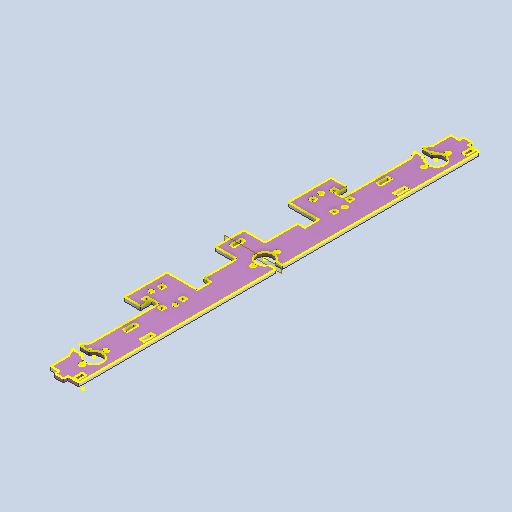
# Autodesk Inventor part: chassis_1_1-03
Saved by Autodesk Inventor 2022 (Build 260153000, 153)
## iProperties
Created: 2023-03-24
Part Number: chassis_1_1-03
Material: 一般
Document SubType Name: Modeling
Designer: Johnny Jou
Density: 79.16 g/cm^3
Appearance: 預設
Mass: 1181.55 g
Surface Area: 130.252 cm^2
Volume: 14.9262 cm^3
Author: Johnny Jou
Autodesk Inventor part; units mm, degrees
ref_plane "YZ Plane" through (0, 0, 0) normal (1, 0, 0) x (0, 1, 0)
ref_plane "XZ Plane" through (0, 0, 0) normal (0, 1, 0) x (-1, 0, 0)
ref_plane "XY Plane" through (0, 0, 0) normal (0, 0, 1) x (1, 0, 0)
sketch "草圖1" plane through (0, 0, 0) normal (0, 1, 0) x (-1, 0, 0)
  line L0 (0, 0) -> (0, -290)
  arc A0 (15, -157.4599) -> (15, -132.5401) centre (16, -145) ccw
  circle A1 centre (16, -145) radius 26 construction
  line L1 (15, -280) -> (15, -157.4599)
  line L2 (15, -132.5401) -> (15, -10)
  circle A2 centre (16, -136.5) radius 1.5
  circle A3 centre (16, -153.5) radius 1.5
  line L3 (20, 0) -> (20, -10)
  line L4 (20, -10) -> (15, -10)
  line L5 (0, -10) -> (0, 0)
  line L6 (6, 0) -> (6, -3)
  line L7 (6, -3) -> (14, -3)
  line L8 (14, -3) -> (14, 0)
  line L9 (0, 0) -> (6, 0)
  line L10 (14, 0) -> (20, 0)
  line L11 (15, 0) -> (14, 0)
  line L12 (6, 0) -> (0, 0)
  line L13 (20, -290) -> (20, -280)
  line L14 (20, -280) -> (15, -280)
  line L15 (0, -290) -> (0, -290)
  line L16 (6, -290) -> (6, -287)
  line L17 (6, -287) -> (14, -287)
  line L18 (14, -287) -> (14, -290)
  line L19 (0, -290) -> (6, -290)
  line L20 (14, -290) -> (20, -290)
  dimension "d1" = 15
  dimension "d2" = 25
  dimension "d3" = 52
  dimension "d4" = 16
  dimension "d6" = 3
  dimension "d7" = 17
  dimension "d8" = 8.5
  dimension "d9" = 10
  dimension "d10" = 20
  dimension "d11" = 8
  dimension "d12" = 3
  dimension "d13" = 6
  dimension "d15" = 3
  dimension "d16" = 8
  dimension "d17" = 6
  dimension "d34" = 290
  dimension "d35" = 145
  dimension "d36" = 10
  dimension "d55" = 8.5
  dimension "d56" = 15
  dimension "d57" = 15
  constraints: 42 end point, 10 parallel, 6 horizontal, 6 perpendicular, 4 centre point, 2 coincident, 2 collinear, 2 point on circle, 1 equal radius, 1 vertical alignment
  measures "d1" distance of L11.start L0.start
  measures "d2" diameter of A0
  measures "d3" diameter of A1
  measures "d4" distance from line of L0 A0.centre
  measures "d6" diameter of A2
  measures "d7" distance of A3.centre A2.centre
  measures "d8" distance of A0.centre A3.centre
  measures "d9" distance of L3.start L3.end
  measures "d10" distance between parallel lines of L0 L3
  measures "d11" distance of L6.end L7.end
  measures "d12" distance of L7.end L8.end
  measures "d13" distance between parallel lines of L5 L6
  measures "d15" distance of L17.end L18.end
  measures "d16" distance of L16.end L17.end
  measures "d17" distance between parallel lines of L0 L16
  measures "d34" distance of L0.start L0.end
  measures "d35" distance from line of L19 A0.centre
  measures "d36" distance of L13.start L13.end
  measures "d55" distance of A0.centre A2.centre
  measures "d56" distance between parallel lines of L0 L1
  measures "d57" distance between parallel lines of L0 L2
extrude "擠出1" add sketch "草圖1" along normal blind 3
sketch "草圖2" plane through (0, 3, 0) normal (0, 1, 0) x (1, 0, 0)
  line L0 (-5, 197) -> (-2, 197)
  line L1 (-2, 197) -> (-2, 205)
  line L2 (-2, 205) -> (-5, 205)
  line L3 (-5, 205) -> (-5, 197)
  arc A0 (-15, 157.4599) -> (-15, 132.5401) centre (-16, 145) ccw projected
  line L4 (-15, 132.5401) -> (-15, 10) projected
  circle A1 centre (-16, 145) radius 12.5 construction
  line L5 (0, 0) -> (0, 290) projected
  line L6 (-11, 4) -> (-8, 4)
  line L7 (-8, 4) -> (-8, 10)
  line L8 (-8, 10) -> (-11, 10)
  line L9 (-11, 10) -> (-11, 4)
  line L10 (-14, 3) -> (-6, 3) projected
  line L11 (-11, 280) -> (-8, 280)
  line L12 (-8, 280) -> (-8, 286)
  line L13 (-8, 286) -> (-11, 286)
  line L14 (-11, 286) -> (-11, 280)
  line L15 (-6, 287) -> (-14, 287) projected
  line L16 (-5, 85) -> (-2, 85)
  line L17 (-2, 85) -> (-2, 93)
  line L18 (-2, 93) -> (-5, 93)
  line L19 (-5, 93) -> (-5, 85)
  line L20 (-15, 280) -> (-15, 157.4599) projected
  line L21 (-13, 129) -> (-5, 129)
  line L22 (-5, 129) -> (-5, 132)
  line L23 (-5, 132) -> (-13, 132)
  line L24 (-13, 132) -> (-13, 129)
  line L25 (-13, 158) -> (-5, 158)
  line L26 (-5, 158) -> (-5, 161)
  line L27 (-5, 161) -> (-13, 161)
  line L28 (-13, 161) -> (-13, 158)
  line L29 (-11, 51) -> (-8, 51)
  line L30 (-8, 51) -> (-8, 59)
  line L31 (-8, 59) -> (-11, 59)
  line L32 (-11, 59) -> (-11, 51)
  line L33 (-11, 55) -> (-8, 55) construction
  line L34 (-11, 231) -> (-8, 231)
  line L35 (-8, 231) -> (-8, 239)
  line L36 (-8, 239) -> (-11, 239)
  line L37 (-11, 239) -> (-11, 231)
  line L38 (-11, 235) -> (-8, 235) construction
  dimension "d20" = 8
  dimension "d21" = 3
  dimension "d22" = 60
  dimension "d23" = 2
  dimension "d24" = 6
  dimension "d25" = 3
  dimension "d27" = 1
  dimension "d28" = 6
  dimension "d29" = 3
  dimension "d31" = 1
  dimension "d58" = 3
  dimension "d59" = 8
  dimension "d60" = 60
  dimension "d69" = 4
  dimension "d70" = 4
  dimension "d104" = 13
  dimension "d106" = 13
  dimension "d108" = 90
  dimension "d109" = 90
  constraints: 68 end point, 16 parallel, 8 equal length, 8 horizontal, 8 perpendicular, 5 collinear, 4 midpoint, 1 coincident, 3 other
  measures "d20" distance of L2.end L0.start
  measures "d21" distance of L1.end L2.end
  measures "d22" distance from line of A0.centre L2
  measures "d23" distance between parallel lines of L5 L1
  measures "d24" distance of L8.end L6.start
  measures "d25" distance of L7.end L8.end
  measures "d27" distance between parallel lines of L10 L6
  measures "d28" distance of L13.end L11.start
  measures "d29" distance of L11.start L11.end
  measures "d31" distance between parallel lines of L15 L13
  measures "d58" distance of L17.end L18.end
  measures "d59" distance of L16.end L17.end
  measures "d60" distance from line of A0.centre L16
  measures "d69" distance between parallel lines of L20 L14
  measures "d70" distance between parallel lines of L4 L9
  measures "d104" distance from line of A0.centre L23
  measures "d106" distance from line of L25 A0.centre
  measures "d108" distance from line of A0.centre L33
  measures "d109" distance from line of A0.centre L38
extrude "擠出2" cut sketch "草圖2" against normal up to surface (3 mm away) contours L9 L8 L7 L6 | L14 L13 L12 L11 | L32 L31 L30 L29 | L37 L36 L35 L34
sketch "草圖3" plane through (0, 3, 0) normal (0, 1, 0) x (1, 0, 0)
  arc A0 (-15, 157.4599) -> (-15, 132.5401) centre (-16, 145) ccw projected
  circle A1 centre (-16, 145) radius 6
  point P0 (0, 0)
  dimension "d37" = 12
  constraints: 1 centre point, 1 coincident
  measures "d37" diameter of A1
extrude "擠出3" cut sketch "草圖3" against normal up to surface (3 mm away)
sketch "草圖4" plane through (0, 3, 0) normal (0, 1, 0) x (1, 0, 0)
  circle A0 centre (-16, 145) radius 6 projected
  arc A1 (-15, 157.4599) -> (-15, 132.5401) centre (-16, 145) ccw projected
  circle A2 centre (-16, 136.5) radius 1.5 projected
  circle A3 centre (-16, 153.5) radius 1.5 projected
  circle A4 centre (-16, 23.5) radius 12.5
  circle A5 centre (-16, 23.5) radius 6
  circle A6 centre (-16, 32) radius 1.5
  circle A7 centre (-16, 15) radius 1.5
  line L0 (-15, 132.5401) -> (-15, 10) projected
  circle A8 centre (-16, 266.5) radius 12.5
  circle A9 centre (-16, 266.5) radius 6
  circle A10 centre (-16, 275) radius 1.5
  circle A11 centre (-16, 258) radius 1.5
  point P0 (0, 0)
  point P1 (-15, 11.0401)
  point P2 (-15, 35.9599)
  dimension "d40" = 3
  dimension "d41" = 12
  dimension "d42" = 25
  dimension "d43" = 17
  dimension "d44" = 8.5
  dimension "d45" = 121.5
  dimension "d48" = 243
  constraints: 8 centre point, 3 vertical alignment, 2 coincident, 1 equal radius, 1 vertical, 8 other
  measures "d40" diameter of A6
  measures "d41" diameter of A5
  measures "d42" diameter of A4
  measures "d43" distance of A7.centre A6.centre
  measures "d44" distance of A4.centre A6.centre
  measures "d45" distance of A0.centre A4.centre
  measures "d48" distance of A4.centre A8.centre
extrude "擠出4" add sketch "草圖4" against normal up to surface (3 mm away) contours A4 L0 A7 A5 A6 | L0 A6 A5 A7 A4 | A8
sketch "草圖6" plane through (0, 3, 0) normal (0, 1, 0) x (1, 0, 0)
  arc A0 (-15, 29.4161) -> (-15, 17.5839) centre (-16, 23.5) ccw projected
  arc A1 (-15, 272.4161) -> (-15, 260.5839) centre (-16, 266.5) ccw projected
  line L0 (-15, 272.4161) -> (-15, 260.5839) projected
  circle A2 centre (-16, 266.5) radius 6
  line L1 (-15, 29.4161) -> (-15, 17.5839) projected
  circle A3 centre (-16, 23.5) radius 6
  point P0 (0, 0)
  point P1 (-15, 260.5839)
  point P2 (-15, 29.4161)
  constraints: 2 coincident, 6 other
extrude "擠出" cut sketch "草圖6" against normal up to surface (3 mm away) contours A3 L1 | L0 A1 | A2 L0
sketch "草圖8" plane through (0, 3, 0) normal (0, 1, 0) x (1, 0, 0)
  circle A0 centre (-16, 266.5) radius 6 projected
  circle A1 centre (-16, 23.5) radius 6 projected
  line L0 (-15, 259.118) -> (-15, 256.882) projected
  arc A2 (-15, 259.118) -> (-15, 256.882) centre (-16, 258) ccw projected
  line L1 (0, 0) -> (0, 290) projected
  line L2 (-6, 290) -> (-6, 287) projected
  line L3 (-6, 287) -> (-14, 287) projected
  line L4 (-14, 287) -> (-14, 290) projected
  line L5 (-14, 290) -> (-20, 290) projected
  line L6 (-20, 290) -> (-20, 280) projected
  line L7 (-20, 280) -> (-15, 280) projected
  line L8 (-15, 280) -> (-15, 278.9599) projected
  arc A3 (-15, 278.9599) -> (-15, 254.0401) centre (-16, 266.5) ccw projected
  line L9 (-15, 254.0401) -> (-15, 157.4599) projected
  arc A4 (-15, 157.4599) -> (-15, 132.5401) centre (-16, 145) ccw projected
  line L10 (-15, 132.5401) -> (-15, 35.9599) projected
  arc A5 (-15, 35.9599) -> (-15, 11.0401) centre (-16, 23.5) ccw projected
  line L11 (-20, 10) -> (-20, 0) projected
  line L12 (-20, 0) -> (-14, 0) projected
  line L13 (-14, 0) -> (-14, 3) projected
  line L14 (-14, 3) -> (-6, 3) projected
  line L15 (-6, 3) -> (-6, 0) projected
  arc A6 (-15, 33.118) -> (-15, 30.882) centre (-16, 32) ccw projected
  line L16 (-15, 33.118) -> (-15, 30.882) projected
  circle A7 centre (-16, 145) radius 6 projected
  line L17 (-8, 286) -> (-8, 280) projected
  line L18 (-8, 280) -> (-11, 280) projected
  line L19 (-11, 280) -> (-11, 286) projected
  line L20 (-11, 286) -> (-8, 286) projected
  line L21 (-8, 4) -> (-11, 4) projected
  line L22 (-11, 4) -> (-11, 10) projected
  line L23 (-8, 10) -> (-8, 4) projected
  circle A8 centre (-16, 136.5) radius 1.5 projected
  circle A9 centre (-16, 153.5) radius 1.5 projected
  arc A10 (-15, 276.118) -> (-15, 273.882) centre (-16, 275) ccw projected
  line L24 (-15, 276.118) -> (-15, 273.882) projected
  circle A11 centre (-20, 40.5367) radius 5
  line L25 (-15, 132.5401) -> (-15, 35.9599) projected
  circle A12 centre (-22.4706, 10) radius 2.4706
  circle A13 centre (-20, 127.9633) radius 5
  circle A14 centre (-20, 162.0367) radius 5
  circle A15 centre (-20, 249.4633) radius 5
  arc A16 (-15, 35.9599) -> (-15, 11.0401) centre (-16, 23.5) ccw projected
  line L26 (-20, 10) -> (-20, 0) projected
  arc A17 (-15, 157.4599) -> (-15, 132.5401) centre (-16, 145) ccw projected
  line L27 (-15, 254.0401) -> (-15, 157.4599) projected
  circle A18 centre (-22.4706, 280) radius 2.4706
  line L28 (-20, 290) -> (-20, 280) projected
  line L29 (-11, 10) -> (-8, 10) projected
  line L30 (-15, 11.0401) -> (-15, 10) projected
  line L31 (-15, 10) -> (-20, 10) projected
  line L32 (0, 290) -> (-6, 290) projected
  line L33 (-6, 0) -> (0, 0) projected
  point P0 (-21.4028, 277.7721)
  point P1 (-18.8571, 254.3309)
  point P2 (-15, 249.4633)
  point P3 (-15, 162.0367)
  point P4 (-18.8571, 157.1691)
  point P5 (-18.8571, 132.8309)
  point P6 (-15, 127.9633)
  point P7 (-15, 40.5367)
  point P8 (-18.8571, 35.6691)
  point P9 (-21.4028, 12.2279)
  point P10 (-20, 9.6573)
  point P11 (-20, 4.6573)
  point P12 (-27.9283, 17.763)
  dimension "d71" = 10
  constraints: 8 tangent, 4 centre point, 3 equal radius, 2 vertical, 8 other
  measures "d71" diameter of A11
extrude "擠出6" add sketch "草圖8" against normal up to surface (3 mm away) contours A12 A5 L30 L31 | L7 L8 A3 A18 | A11 L10 A5 | A3 L9 A15 | A13 A4 L10 | L9 A4 A14
sketch "草圖9" plane through (0, 3, 0) normal (0, 1, 0) x (1, 0, 0)
  circle A0 centre (-16, 266.5) radius 6 projected
  circle A1 centre (-16, 23.5) radius 6 projected
  line L0 (-15, 259.118) -> (-15, 256.882) projected
  arc A2 (-15, 259.118) -> (-15, 256.882) centre (-16, 258) ccw projected
  line L1 (0, 0) -> (0, 290) projected
  line L2 (-6, 290) -> (-6, 287) projected
  line L3 (-6, 287) -> (-14, 287) projected
  line L4 (-14, 287) -> (-14, 290) projected
  line L5 (-14, 290) -> (-20, 290) projected
  line L6 (-20, 290) -> (-20, 280) projected
  arc A3 (-21.4028, 277.7721) -> (-20, 280) centre (-22.4706, 280) ccw projected
  arc A4 (-21.4028, 277.7721) -> (-18.8571, 254.3309) centre (-16, 266.5) ccw projected
  arc A5 (-15, 249.4633) -> (-18.8571, 254.3309) centre (-20, 249.4633) ccw projected
  line L7 (-15, 249.4633) -> (-15, 162.0367) projected
  arc A6 (-18.8571, 157.1691) -> (-15, 162.0367) centre (-20, 162.0367) ccw projected
  arc A7 (-18.8571, 157.1691) -> (-18.8571, 132.8309) centre (-16, 145) ccw projected
  arc A8 (-15, 127.9633) -> (-18.8571, 132.8309) centre (-20, 127.9633) ccw projected
  line L8 (-15, 127.9633) -> (-15, 40.5367) projected
  arc A9 (-18.8571, 35.6691) -> (-15, 40.5367) centre (-20, 40.5367) ccw projected
  arc A10 (-18.8571, 35.6691) -> (-21.4028, 12.2279) centre (-16, 23.5) ccw projected
  arc A11 (-20, 10) -> (-21.4028, 12.2279) centre (-22.4706, 10) ccw projected
  line L9 (-20, 10) -> (-20, 0) projected
  line L10 (-20, 0) -> (-14, 0) projected
  line L11 (-14, 0) -> (-14, 3) projected
  line L12 (-14, 3) -> (-6, 3) projected
  line L13 (-6, 3) -> (-6, 0) projected
  arc A12 (-15, 33.118) -> (-15, 30.882) centre (-16, 32) ccw projected
  line L14 (-15, 33.118) -> (-15, 30.882) projected
  circle A13 centre (-16, 145) radius 6 projected
  line L15 (-8, 286) -> (-8, 280) projected
  line L16 (-8, 280) -> (-11, 280) projected
  line L17 (-11, 280) -> (-11, 286) projected
  line L18 (-11, 286) -> (-8, 286) projected
  line L19 (-8, 4) -> (-11, 4) projected
  line L20 (-11, 4) -> (-11, 10) projected
  line L21 (-8, 10) -> (-8, 4) projected
  circle A14 centre (-16, 136.5) radius 1.5 projected
  circle A15 centre (-16, 153.5) radius 1.5 projected
  arc A16 (-15, 276.118) -> (-15, 273.882) centre (-16, 275) ccw projected
  line L22 (-15, 276.118) -> (-15, 273.882) projected
  arc A17 (-15, 16.118) -> (-15, 13.882) centre (-16, 15) ccw projected
  circle A18 centre (-16, 15) radius 1.5
  line L23 (-15, 33.118) -> (-15, 30.882) projected
  circle A19 centre (-16, 32) radius 1.5
  circle A20 centre (-16, 258) radius 1.5
  circle A21 centre (-16, 275) radius 1.5
  line L24 (-28.5, 264) -> (-21.4544, 264)
  line L25 (-21.4544, 264) -> (-21.4544, 269)
  line L26 (-21.4544, 269) -> (-28.5, 269)
  line L27 (-28.5, 269) -> (-28.5, 264)
  circle A22 centre (-16, 266.5) radius 6 projected
  arc A23 (-21.4028, 277.7721) -> (-18.8571, 254.3309) centre (-16, 266.5) ccw projected
  line L28 (-28.5, 142.5) -> (-21.4544, 142.5)
  line L29 (-21.4544, 142.5) -> (-21.4544, 147.5)
  line L30 (-21.4544, 147.5) -> (-28.5, 147.5)
  line L31 (-28.5, 147.5) -> (-28.5, 142.5)
  circle A24 centre (-16, 145) radius 6 projected
  line L32 (-28.5, 21) -> (-21.4544, 21)
  line L33 (-21.4544, 21) -> (-21.4544, 26)
  line L34 (-21.4544, 26) -> (-28.5, 26)
  line L35 (-28.5, 26) -> (-28.5, 21)
  arc A25 (-18.8571, 35.6691) -> (-21.4028, 12.2279) centre (-16, 23.5) ccw projected
  circle A26 centre (-16, 23.5) radius 6 projected
  line L36 (-11, 10) -> (-8, 10) projected
  line L37 (-15, 16.118) -> (-15, 13.882) projected
  arc A27 (-15, 16.118) -> (-15, 13.882) centre (-16, 15) ccw projected
  line L38 (0, 290) -> (-6, 290) projected
  line L39 (-6, 0) -> (0, 0) projected
  circle A28 centre (-16, 145) radius 6 projected
  line L40 (0, 0) -> (0, 290) projected
  line L41 (-10.5456, 142.5) -> (0, 142.5)
  line L42 (0, 142.5) -> (0, 147.5)
  line L43 (0, 147.5) -> (-10.5456, 147.5)
  line L44 (-10.5456, 147.5) -> (-10.5456, 142.5)
  point P0 (-28.2474, 269)
  point P1 (-28.2474, 264)
  point P2 (-28.2474, 147.5)
  point P3 (-28.2474, 142.5)
  point P4 (-28.2474, 26)
  point P5 (-28.2474, 21)
  point P6 (-15, 30.882)
  point P7 (-21.8029, 14.9747)
  point P8 (-20.38, 12.3993)
  point P9 (-21.4544, 19)
  point P10 (-21.4544, 14.5244)
  point P11 (0, 147.5)
  point P12 (-10.5456, 147.5)
  point P13 (0, 142.5)
  dimension "d74" = 5
  dimension "d75" = 5
  dimension "d76" = 5
  constraints: 32 end point, 8 parallel, 4 coincident, 4 horizontal, 4 perpendicular, 3 point on circle, 3 tangent, 2 collinear, 1 point on line, 20 other
  measures "d74" distance of L26.end L24.start
  measures "d75" distance of L30.end L28.start
  measures "d76" distance of L34.end L32.start
extrude "擠出7" cut sketch "草圖9" against normal up to surface (3 mm away) contours A0 L24 A4 L26 | L43 L1 L41 A13 | L34 A1 L32 A10 | A10 L35 L34 | A10 L32 L35 | A20 L0 | A19 L14 | A21 L22 | L37 A17 | A18 L37
fillet "圓角1" radius 0.5 8 edges at (-21.4544, 1.5, -269) (-28.2474, 1.5, -269) (-21.4544, 1.5, -264) (-28.2474, 1.5, -264) (-21.4544, 1.5, -26) (-28.2474, 1.5, -26) (-28.2474, 1.5, -21) (-21.4544, 1.5, -21)
sketch "草圖11" plane through (0, 3, 0) normal (0, 1, 0) x (1, 0, 0)
  line L0 (-15, 127.9633) -> (-15, 40.5367) projected
  line L1 (-15, 249.4633) -> (-15, 162.0367) projected
  line L2 (-28.5, 242.5) -> (-15, 242.5)
  line L3 (-28.5, 245.5) -> (-28.5, 242.5)
  line L4 (-33.5, 242.5) -> (-28.5, 245.5)
  line L5 (-15, 227.5) -> (-28.5, 227.5)
  line L6 (-28.5, 227.5) -> (-28.5, 224.5)
  line L7 (-33.5, 227.5) -> (-33.5, 242.5)
  line L8 (-28.5, 224.5) -> (-33.5, 227.5)
  arc A0 (-21.3227, 263.7308) -> (-21.3227, 269.2692) centre (-16, 266.5) ccw projected
  arc A1 (-10.5456, 147.5) -> (-10.5456, 142.5) centre (-16, 145) ccw projected
  line L9 (-16, 145) -> (0, 145)
  line L10 (-28.5, 47.5) -> (-15, 47.5)
  line L11 (-28.5, 44.5) -> (-28.5, 47.5)
  line L12 (-33.5, 47.5) -> (-28.5, 44.5)
  line L13 (-15, 62.5) -> (-28.5, 62.5)
  line L14 (-28.5, 62.5) -> (-28.5, 65.5)
  line L15 (-33.5, 62.5) -> (-33.5, 47.5)
  line L16 (-28.5, 65.5) -> (-33.5, 62.5)
  line L17 (-28, 245.5) -> (-15, 245.5)
  line L18 (-15, 245.5) -> (-15, 242.5)
  line L19 (-15, 242.5) -> (-19.5, 242.5)
  line L20 (-28, 243) -> (-28, 245.5)
  line L21 (-15, 227.5) -> (-19.5, 227.5)
  line L22 (-28, 227) -> (-28, 224.5)
  line L23 (-28, 224.5) -> (-15, 224.5)
  line L24 (-15, 224.5) -> (-15, 227.5)
  line L25 (-19.5, 242.5) -> (-27.5, 242.5)
  line L26 (-27.5, 242.5) -> (-27.5, 243)
  line L27 (-27.5, 243) -> (-28, 243)
  line L28 (-19.5, 227.5) -> (-27.5, 227.5)
  line L29 (-27.5, 227.5) -> (-27.5, 227)
  line L30 (-27.5, 227) -> (-28, 227)
  line L31 (-28, 47) -> (-28, 44.5)
  line L32 (-28, 44.5) -> (-15, 44.5)
  line L33 (-27.5, 47.5) -> (-27.5, 47)
  line L34 (-27.5, 47) -> (-28, 47)
  line L35 (-28, 65.5022) -> (-15, 65.5022)
  line L36 (-28, 63.0022) -> (-28, 65.5022)
  line L37 (-27.5, 62.5) -> (-27.5, 63)
  line L38 (-27.5, 63) -> (-28, 63.0022)
  arc A2 (-21.3227, 20.7308) -> (-21.3227, 26.2692) centre (-16, 23.5) ccw projected
  line L39 (-15, 54) -> (-15, 62)
  line L40 (-8, 51) -> (-11, 51) projected
  line L41 (-11, 59) -> (-8, 59) projected
  line L42 (-15, 234) -> (-15, 242)
  line L43 (-8, 231) -> (-11, 231) projected
  line L44 (-11, 239) -> (-8, 239) projected
  line L45 (-22.9, 239) -> (-20, 239)
  line L46 (-20, 239) -> (-20, 231)
  line L47 (-20, 231) -> (-22.9, 231)
  line L48 (-22.9, 231) -> (-22.9, 239)
  line L49 (-8, 239) -> (-11, 239) projected
  line L50 (-11, 231) -> (-8, 231) projected
  line L51 (-11, 239) -> (-11, 231) projected
  line L52 (-22.9, 59) -> (-20, 59)
  line L53 (-20, 59) -> (-20, 51)
  line L54 (-20, 51) -> (-22.9, 51)
  line L55 (-22.9, 51) -> (-22.9, 59)
  line L56 (-8, 59) -> (-11, 59) projected
  line L57 (-11, 51) -> (-8, 51) projected
  line L58 (-11, 59) -> (-11, 51) projected
  point P0 (0, 0)
  point P1 (-22, 148)
  point P2 (-22, 148)
  point P3 (-15, 47.5)
  point P4 (-15, 62.5)
  point P5 (-15, 245.5)
  point P6 (-15, 224.5)
  dimension "d2" = 25
  dimension "d80" = 15
  dimension "d81" = 3
  dimension "d82" = 13.5
  dimension "d83" = 3
  dimension "d84" = 13.5
  dimension "d85" = 24
  dimension "d88" = 5
  dimension "d89" = 0.5
  dimension "d90" = 0.5
  dimension "d91" = 0.5
  dimension "d92" = 0.5
  dimension "d93" = 0.5
  dimension "d94" = 0.5
  dimension "d95" = 0.5
  dimension "d96" = 0.5
  dimension "d97" = 3
  dimension "d98" = 3
  dimension "d99" = 0.5
  dimension "d100" = 0.5
  dimension "d101" = 13
  dimension "d102" = 2.5
  dimension "d103" = 0.5
  dimension "d121" = 2.9
  dimension "d122" = 9
  dimension "d123" = 2.9
  dimension "d124" = 9
  constraints: 94 end point, 11 horizontal, 10 parallel, 8 symmetric about line, 7 vertical, 6 collinear, 6 perpendicular, 6 point on line, 3 horizontal alignment
  measures "d80" distance of L7.start L4.start
  measures "d81" distance of L5.end L6.end
  measures "d82" distance of L5.start L5.end
  measures "d83" distance of L3.start L2.start
  measures "d84" distance of L2.start L2.end
  measures "d85" distance from line of A0.centre L2
  measures "d88" distance between parallel lines of L3 L7
  measures "d89" distance between parallel lines of L3 L20
  measures "d90" distance between parallel lines of L6 L22
  measures "d91" distance of L20.start L26.end
  measures "d92" distance of L25.end L26.end
  measures "d93" distance of L34.start L31.start
  measures "d94" distance of L33.start L34.start
  measures "d95" distance of L28.end L29.end
  measures "d96" distance of L29.end L22.start
  measures "d97" distance between parallel lines of L23 L5
  measures "d98" distance between parallel lines of L10 L32
  measures "d99" distance of L38.end L37.end
  measures "d100" distance of L37.start L37.end
  measures "d101" distance of L36.end L35.end
  measures "d102" distance of L38.end L36.end
  measures "d103" distance between parallel lines of L11 L31
  measures "d121" distance between parallel lines of L46 L48
  measures "d122" distance between parallel lines of L51 L46
  measures "d123" distance between parallel lines of L53 L55
  measures "d124" distance between parallel lines of L58 L53
extrude "擠出8" add sketch "草圖11" against normal up to surface (3 mm away)
fillet "圓角2" radius 2 4 edges at (-15, 1.5, -44.5) (-15, 1.5, -65.5022) (-15, 1.5, -224.5) (-15, 1.5, -245.5)
sketch "草圖15" plane through (0, 3, 0) normal (0, 1, 0) x (1, 0, 0)
  line L0 (0, 290) -> (-6, 290) projected
  line L1 (0, 0) -> (-6, 0)
  line L2 (-6, 0) -> (-6, 290)
  line L3 (-6, 290) -> (0, 290)
  line L4 (0, 290) -> (0, 0)
  line L5 (-6, 290) -> (-6, 287) projected
  constraints: 8 end point, 2 parallel, 1 collinear, 1 horizontal, 1 perpendicular, 1 point on line
extrude "擠出10" cut sketch "草圖15" against normal up to surface (3 mm away)
sketch "草圖17" plane through (0, 0, 0) normal (0, -1, 0) x (1, 0, 0)
  line L0 (-26, -287) -> (-20, -287)
  line L1 (-20, -287) -> (-20, -274)
  line L2 (-20, -274) -> (-26, -274)
  line L3 (-26, -274) -> (-26, -287)
  line L4 (-6, -287) -> (-14, -287) projected
  line L5 (-20, -290) -> (-20, -280) projected
  arc A0 (-28.1031, -269.625) -> (-21.4028, -277.7721) centre (-16, -266.5) ccw projected
  circle A1 centre (-16, -15) radius 1.5 projected
  circle A2 centre (-16, -32) radius 1.5 projected
  circle A3 centre (-16, -275) radius 1.5 projected
  circle A4 centre (-16, -258) radius 1.5 projected
  circle A5 centre (-16, -153.5) radius 1.5 projected
  circle A6 centre (-16, -136.5) radius 1.5 projected
  line L6 (-11, -280) -> (-8, -280) projected
  line L7 (-8, -280) -> (-8, -286) projected
  line L8 (-8, -286) -> (-11, -286) projected
  line L9 (-11, -286) -> (-11, -280) projected
  line L10 (-8, -231) -> (-8, -239) projected
  line L11 (-8, -239) -> (-11, -239) projected
  line L12 (-11, -239) -> (-11, -231) projected
  line L13 (-11, -231) -> (-8, -231) projected
  line L14 (-8, -4) -> (-8, -10) projected
  line L15 (-8, -10) -> (-11, -10) projected
  line L16 (-11, -10) -> (-11, -4) projected
  line L17 (-11, -4) -> (-8, -4) projected
  line L18 (-11, -51) -> (-8, -51) projected
  line L19 (-8, -51) -> (-8, -59) projected
  line L20 (-8, -59) -> (-11, -59) projected
  line L21 (-11, -59) -> (-11, -51) projected
  line L22 (-6, -142.5) -> (-6, -3) projected
  line L23 (-14, -3) -> (-6, -3) projected
  line L24 (-14, 0) -> (-14, -3) projected
  line L25 (-20, 0) -> (-14, 0) projected
  line L26 (-20, -10) -> (-20, 0) projected
  arc A7 (-21.4028, -12.2279) -> (-20, -10) centre (-22.4706, -10) ccw projected
  arc A8 (-21.4028, -12.2279) -> (-28.1031, -20.375) centre (-16, -23.5) ccw projected
  arc A9 (-28.1031, -20.375) -> (-27.619, -21) centre (-27.619, -20.5) ccw projected
  line L27 (-27.619, -21) -> (-21.7663, -21) projected
  arc A10 (-21.7663, -21) -> (-21.3227, -20.7308) centre (-21.7663, -20.5) ccw projected
  arc A11 (-21.3227, -26.2692) -> (-21.3227, -20.7308) centre (-16, -23.5) ccw projected
  arc A12 (-21.3227, -26.2692) -> (-21.7663, -26) centre (-21.7663, -26.5) ccw projected
  line L28 (-21.7663, -26) -> (-27.619, -26) projected
  arc A13 (-27.619, -26) -> (-28.1031, -26.625) centre (-27.619, -26.5) ccw projected
  arc A14 (-28.1031, -26.625) -> (-18.8571, -35.6691) centre (-16, -23.5) ccw projected
  arc A15 (-15, -40.5367) -> (-18.8571, -35.6691) centre (-20, -40.5367) ccw projected
  line L29 (-15, -42.5) -> (-15, -40.5367) projected
  arc A16 (-17, -44.5) -> (-15, -42.5) centre (-17, -42.5) ccw projected
  line L30 (-17, -44.5) -> (-28, -44.5) projected
  line L31 (-28, -44.5) -> (-28, -47) projected
  line L32 (-28, -47) -> (-27.5, -47) projected
  line L33 (-27.5, -47) -> (-27.5, -47.5) projected
  line L34 (-27.5, -47.5) -> (-28.5, -47.5) projected
  line L35 (-28.5, -47.5) -> (-28.5, -44.5) projected
  line L36 (-28.5, -44.5) -> (-33.5, -47.5) projected
  line L37 (-33.5, -47.5) -> (-33.5, -62.5) projected
  line L38 (-33.5, -62.5) -> (-28.5, -65.5) projected
  line L39 (-28.5, -65.5) -> (-28.5, -62.5) projected
  line L40 (-28.5, -62.5) -> (-27.5, -62.5) projected
  line L41 (-27.5, -62.5) -> (-27.5, -63) projected
  line L42 (-27.5, -63) -> (-28, -63.0022) projected
  line L43 (-28, -63.0022) -> (-28, -65.5022) projected
  line L44 (-28, -65.5022) -> (-17, -65.5022) projected
  arc A17 (-15, -67.5022) -> (-17, -65.5022) centre (-17, -67.5022) ccw projected
  line L45 (-15, -127.9633) -> (-15, -67.5022) projected
  arc A18 (-18.8571, -132.8309) -> (-15, -127.9633) centre (-20, -127.9633) ccw projected
  arc A19 (-18.8571, -132.8309) -> (-18.8571, -157.1691) centre (-16, -145) ccw projected
  arc A20 (-10.5456, -142.5) -> (-10.5456, -147.5) centre (-16, -145) ccw projected
  arc A21 (-15, -162.0367) -> (-18.8571, -157.1691) centre (-20, -162.0367) ccw projected
  line L46 (-15, -222.5) -> (-15, -162.0367) projected
  arc A22 (-17, -224.5) -> (-15, -222.5) centre (-17, -222.5) ccw projected
  line L47 (-17, -224.5) -> (-28, -224.5) projected
  line L48 (-28, -224.5) -> (-28, -227) projected
  line L49 (-28, -227) -> (-27.5, -227) projected
  line L50 (-27.5, -227) -> (-27.5, -227.5) projected
  line L51 (-27.5, -227.5) -> (-28.5, -227.5) projected
  line L52 (-28.5, -227.5) -> (-28.5, -224.5) projected
  line L53 (-28.5, -224.5) -> (-33.5, -227.5) projected
  line L54 (-33.5, -227.5) -> (-33.5, -242.5) projected
  line L55 (-33.5, -242.5) -> (-28.5, -245.5) projected
  line L56 (-28.5, -245.5) -> (-28.5, -242.5) projected
  line L57 (-28.5, -242.5) -> (-27.5, -242.5) projected
  line L58 (-27.5, -242.5) -> (-27.5, -243) projected
  line L59 (-27.5, -243) -> (-28, -243) projected
  line L60 (-28, -243) -> (-28, -245.5) projected
  line L61 (-28, -245.5) -> (-17, -245.5) projected
  arc A23 (-15, -247.5) -> (-17, -245.5) centre (-17, -247.5) ccw projected
  line L62 (-15, -249.4633) -> (-15, -247.5) projected
  arc A24 (-18.8571, -254.3309) -> (-15, -249.4633) centre (-20, -249.4633) ccw projected
  arc A25 (-18.8571, -254.3309) -> (-28.1031, -263.375) centre (-16, -266.5) ccw projected
  arc A26 (-28.1031, -263.375) -> (-27.619, -264) centre (-27.619, -263.5) ccw projected
  line L63 (-27.619, -264) -> (-21.7663, -264) projected
  arc A27 (-21.7663, -264) -> (-21.3227, -263.7308) centre (-21.7663, -263.5) ccw projected
  arc A28 (-21.3227, -269.2692) -> (-21.3227, -263.7308) centre (-16, -266.5) ccw projected
  arc A29 (-21.3227, -269.2692) -> (-21.7663, -269) centre (-21.7663, -269.5) ccw projected
  line L64 (-21.7663, -269) -> (-27.619, -269) projected
  arc A30 (-27.619, -269) -> (-28.1031, -269.625) centre (-27.619, -269.5) ccw projected
  arc A31 (-28.1031, -269.625) -> (-21.4028, -277.7721) centre (-16, -266.5) ccw projected
  arc A32 (-20, -280) -> (-21.4028, -277.7721) centre (-22.4706, -280) ccw projected
  line L65 (-20, -290) -> (-20, -280) projected
  line L66 (-14, -290) -> (-20, -290) projected
  line L67 (-14, -287) -> (-14, -290) projected
  line L68 (-6, -287) -> (-14, -287) projected
  arc A33 (-18.8571, -254.3309) -> (-28.1031, -263.375) centre (-16, -266.5) ccw projected
  line L69 (-26, -259) -> (-26, -245.5)
  line L70 (-17, -245.5) -> (-28, -245.5) projected
  line L71 (-26, -224.5) -> (-26, -149.5)
  arc A34 (-18.8571, -132.8309) -> (-18.8571, -157.1691) centre (-16, -145) ccw projected
  line L72 (-26, -137.5) -> (-26, -65.5022)
  line L73 (-28, -44.5) -> (-17, -44.5) projected
  line L74 (-26, -44.5) -> (-26, -31)
  line L75 (-26, -16) -> (-20, -16)
  line L76 (-20, -16) -> (-20, -3)
  line L77 (-20, -3) -> (-26, -3)
  line L78 (-26, -3) -> (-26, -16)
  line L79 (-14, -3) -> (-6, -3) projected
  line L80 (-20, -10) -> (-20, 0) projected
  line L81 (-6, -287) -> (-6, -147.5) projected
  line L82 (-6, -147.5) -> (-10.5456, -147.5) projected
  line L83 (-10.5456, -142.5) -> (-6, -142.5) projected
  point P0 (0, 0)
  point P1 (-28.1031, -144.875)
  point P2 (-20, -3)
  point P3 (-26, -137.5)
  point P4 (-26, -152.5)
  dimension "d118" = 6
  constraints: 24 end point, 8 collinear, 7 point on line, 5 point on circle, 4 parallel, 2 horizontal, 2 perpendicular
  measures "d118" distance of L0.start L0.end
extrude "擠出11" add sketch "草圖17" against normal up to surface (3 mm away) contours L3 A0 A32 L1 L0 | L69 L61 A23 L62 A24 A25 | L26 A7 A8 L78 L77 | A14 A15 L29 A16 L30 L74 | L71 A19 A21 L46 A22 L47 | L72 L44 A17 L45 A18 A19
sketch "草圖21" plane through (0, 3, 0) normal (0, 1, 0) x (1, 0, 0)
  line L0 (-26, 135) -> (-41, 135)
  line L1 (-41, 135) -> (-41, 155)
  line L2 (-41, 155) -> (-26, 155)
  line L3 (-26, 155) -> (-26, 135)
  line L4 (-26, 152.5) -> (-26, 224.5) projected
  arc A0 (-10.5456, 147.5) -> (-10.5456, 142.5) centre (-16, 145) ccw projected
  line L5 (-34.1, 141) -> (-37, 141)
  line L6 (-37, 141) -> (-37, 149)
  line L7 (-37, 149) -> (-34.1, 149)
  line L8 (-34.1, 149) -> (-34.1, 141)
  point P0 (0, 0)
  point P1 (-41, 145)
  point P2 (-37, 145)
  dimension "d137" = 20
  dimension "d138" = 15
  dimension "d141" = 8
  dimension "d142" = 2.9
  dimension "d143" = 4
  constraints: 16 end point, 4 parallel, 2 horizontal, 2 horizontal alignment, 2 midpoint, 2 perpendicular, 1 collinear
  measures "d137" distance between parallel lines of L2 L0
  measures "d138" distance between parallel lines of L3 L1
  measures "d141" distance of L5.end L6.end
  measures "d142" distance of L6.end L7.end
  measures "d143" distance between parallel lines of L1 L6
extrude "擠出13" add sketch "草圖21" against normal up to surface (3 mm away)
sketch "草圖22" plane through (0, 3, 0) normal (0, 1, 0) x (1, 0, 0)
  line L0 (-28, 224.5) -> (-26, 224.5) projected
  line L1 (-26, 245.5) -> (-28, 245.5) projected
  line L2 (-26, 224.5) -> (-26, 245.5)
  line L3 (-26, 31) -> (-26, 44.5) projected
  line L4 (-26, 65.5022) -> (-26, 135) projected
  line L5 (-26, 44.5) -> (-26, 65.5022)
  line L6 (-34.1, 141) -> (-37, 141) projected
  line L7 (-37, 141) -> (-37, 149) projected
  line L8 (-37, 149) -> (-34.1, 149) projected
  line L9 (-34.1, 149) -> (-34.1, 141) projected
  line L10 (-26, 65.5022) -> (-26, 135) projected
  line L11 (-26, 65.5022) -> (-28, 65.5022) projected
  line L12 (-28, 65.5022) -> (-28, 63.0022) projected
  line L13 (-28, 63.0022) -> (-27.5, 63) projected
  line L14 (-27.5, 63) -> (-27.5, 62.5) projected
  line L15 (-27.5, 62.5) -> (-28.5, 62.5) projected
  line L16 (-28.5, 62.5) -> (-28.5, 65.5) projected
  line L17 (-28.5, 65.5) -> (-33.5, 62.5) projected
  line L18 (-33.5, 62.5) -> (-33.5, 47.5) projected
  line L19 (-33.5, 47.5) -> (-28.5, 44.5) projected
  line L20 (-28.5, 44.5) -> (-28.5, 47.5) projected
  line L21 (-28.5, 47.5) -> (-27.5, 47.5) projected
  line L22 (-27.5, 47.5) -> (-27.5, 47) projected
  line L23 (-27.5, 47) -> (-28, 47) projected
  line L24 (-28, 47) -> (-28, 44.5) projected
  line L25 (-28, 44.5) -> (-26, 44.5) projected
  line L26 (-26, 31) -> (-26, 44.5) projected
  arc A0 (-26, 31) -> (-28.1031, 26.625) centre (-16, 23.5) ccw projected
  arc A1 (-28.1031, 26.625) -> (-27.619, 26) centre (-27.619, 26.5) ccw projected
  line L27 (-27.619, 26) -> (-21.7663, 26) projected
  arc A2 (-21.7663, 26) -> (-21.3227, 26.2692) centre (-21.7663, 26.5) ccw projected
  arc A3 (-21.3227, 20.7308) -> (-21.3227, 26.2692) centre (-16, 23.5) ccw projected
  arc A4 (-21.3227, 20.7308) -> (-21.7663, 21) centre (-21.7663, 20.5) ccw projected
  line L28 (-21.7663, 21) -> (-27.619, 21) projected
  arc A5 (-27.619, 21) -> (-28.1031, 20.375) centre (-27.619, 20.5) ccw projected
  arc A6 (-28.1031, 20.375) -> (-26, 16) centre (-16, 23.5) ccw projected
  line L29 (-26, 3) -> (-26, 16) projected
  line L30 (-20, 3) -> (-26, 3) projected
  line L31 (-20, 3) -> (-20, 0) projected
  line L32 (-20, 0) -> (-14, 0) projected
  line L33 (-14, 0) -> (-14, 3) projected
  line L34 (-14, 3) -> (-6, 3) projected
  line L35 (-6, 3) -> (-6, 142.5) projected
  line L36 (-6, 142.5) -> (-10.5456, 142.5) projected
  arc A7 (-10.5456, 147.5) -> (-10.5456, 142.5) centre (-16, 145) ccw projected
  line L37 (-10.5456, 147.5) -> (-6, 147.5) projected
  line L38 (-6, 147.5) -> (-6, 287) projected
  line L39 (-6, 287) -> (-14, 287) projected
  line L40 (-14, 287) -> (-14, 290) projected
  line L41 (-14, 290) -> (-20, 290) projected
  line L42 (-20, 290) -> (-20, 287) projected
  line L43 (-26, 287) -> (-20, 287) projected
  line L44 (-26, 274) -> (-26, 287) projected
  arc A8 (-26, 274) -> (-28.1031, 269.625) centre (-16, 266.5) ccw projected
  arc A9 (-28.1031, 269.625) -> (-27.619, 269) centre (-27.619, 269.5) ccw projected
  line L45 (-27.619, 269) -> (-21.7663, 269) projected
  arc A10 (-21.7663, 269) -> (-21.3227, 269.2692) centre (-21.7663, 269.5) ccw projected
  arc A11 (-21.3227, 263.7308) -> (-21.3227, 269.2692) centre (-16, 266.5) ccw projected
  arc A12 (-21.3227, 263.7308) -> (-21.7663, 264) centre (-21.7663, 263.5) ccw projected
  line L46 (-21.7663, 264) -> (-27.619, 264) projected
  arc A13 (-27.619, 264) -> (-28.1031, 263.375) centre (-27.619, 263.5) ccw projected
  arc A14 (-28.1031, 263.375) -> (-26, 259) centre (-16, 266.5) ccw projected
  line L47 (-26, 245.5) -> (-26, 259) projected
  line L48 (-26, 245.5) -> (-28, 245.5) projected
  line L49 (-28, 245.5) -> (-28, 243) projected
  line L50 (-28, 243) -> (-27.5, 243) projected
  line L51 (-27.5, 243) -> (-27.5, 242.5) projected
  line L52 (-27.5, 242.5) -> (-28.5, 242.5) projected
  line L53 (-28.5, 242.5) -> (-28.5, 245.5) projected
  line L54 (-28.5, 245.5) -> (-33.5, 242.5) projected
  line L55 (-33.5, 242.5) -> (-33.5, 227.5) projected
  line L56 (-33.5, 227.5) -> (-28.5, 224.5) projected
  line L57 (-28.5, 224.5) -> (-28.5, 227.5) projected
  line L58 (-28.5, 227.5) -> (-27.5, 227.5) projected
  line L59 (-27.5, 227.5) -> (-27.5, 227) projected
  line L60 (-27.5, 227) -> (-28, 227) projected
  line L61 (-28, 227) -> (-28, 224.5) projected
  line L62 (-28, 224.5) -> (-26, 224.5) projected
  line L63 (-26, 155) -> (-26, 224.5) projected
  line L64 (-26, 155) -> (-41, 155) projected
  line L65 (-41, 155) -> (-41, 135) projected
  line L66 (-41, 135) -> (-26, 135) projected
  line L67 (-22.9, 239) -> (-20, 239) projected
  line L68 (-20, 239) -> (-20, 231) projected
  line L69 (-20, 231) -> (-22.9, 231) projected
  line L70 (-22.9, 231) -> (-22.9, 239) projected
  line L71 (-22.9, 59) -> (-20, 59) projected
  line L72 (-20, 59) -> (-20, 51) projected
  line L73 (-20, 51) -> (-22.9, 51) projected
  line L74 (-22.9, 51) -> (-22.9, 59) projected
  circle A15 centre (-16, 153.5) radius 1.5 projected
  circle A16 centre (-16, 136.5) radius 1.5 projected
  line L75 (-8, 231) -> (-11, 231) projected
  line L76 (-11, 231) -> (-11, 239) projected
  line L77 (-11, 239) -> (-8, 239) projected
  line L78 (-8, 239) -> (-8, 231) projected
  line L79 (-8, 286) -> (-8, 280) projected
  line L80 (-8, 280) -> (-11, 280) projected
  line L81 (-11, 280) -> (-11, 286) projected
  line L82 (-11, 286) -> (-8, 286) projected
  line L83 (-8, 51) -> (-11, 51) projected
  line L84 (-11, 51) -> (-11, 59) projected
  line L85 (-11, 59) -> (-8, 59) projected
  line L86 (-8, 59) -> (-8, 51) projected
  line L87 (-8, 10) -> (-8, 4) projected
  line L88 (-8, 4) -> (-11, 4) projected
  line L89 (-11, 4) -> (-11, 10) projected
  line L90 (-11, 10) -> (-8, 10) projected
  circle A17 centre (-16, 15) radius 1.5 projected
  circle A18 centre (-16, 275) radius 1.5 projected
  circle A19 centre (-16, 258) radius 1.5 projected
  circle A20 centre (-16, 32) radius 1.5 projected
  point P0 (0, 0)
  constraints: 4 end point, 1 collinear, 1 vertical
extrude "擠出14" cut sketch "草圖22" against normal up to surface (3 mm away) contours L61 L60 L59 L58 L57 L56 L55 L54 L53 L52 L51 L50 L49 L1 L2 L0 | L5 L25 L24 L23 L22 L21 L20 L19 L18 L17 L16 L15 L14 L13 L12 L11
sketch "草圖23" plane through (0, 3, 0) normal (0, 1, 0) x (1, 0, 0)
  line L0 (-26, 65.5022) -> (-26, 135) projected
  line L1 (-26, 71.8144) -> (-42.4222, 71.8144)
  line L2 (-42.4222, 71.8144) -> (-42.4222, 101.8144)
  line L3 (-42.4222, 101.8144) -> (-26, 101.8144)
  line L4 (-26, 101.8144) -> (-26, 71.8144)
  line L5 (-31, 71.8144) -> (-25, 71.8144)
  line L6 (-25, 71.8144) -> (-25, 79.8144)
  line L7 (-25, 79.8144) -> (-31, 79.8144)
  line L8 (-31, 79.8144) -> (-31, 71.8144)
  line L9 (-28, 65.5022) -> (-28, 63.0022) projected
  point P0 (0, 0)
  point P1 (-26, 31)
  point P2 (-28, 79.8144)
  point P3 (-28, 64.2522)
  point P4 (-26, 79.8144)
  point P5 (-26, 101.8144)
  dimension "d146" = 8
  dimension "d147" = 6
  dimension "d148" = 30
  constraints: 16 end point, 4 parallel, 2 horizontal, 2 midpoint, 2 perpendicular, 2 point on line, 1 vertical alignment
  measures "d146" distance of L7.end L5.start
  measures "d147" distance of L6.end L7.end
  measures "d148" distance of L1.end L2.end
extrude "擠出15" add sketch "草圖23" against normal up to surface (3 mm away) contours L7 L8 L1 L2 L3 L0
sketch "草圖24" plane through (0, 3, 0) normal (0, 1, 0) x (1, 0, 0)
  line L0 (-31, 71.8144) -> (-42.4222, 71.8144) projected
  line L1 (-31, 71.8144) -> (-25, 71.8144)
  line L2 (-25, 71.8144) -> (-25, 79.8144)
  line L3 (-25, 79.8144) -> (-31, 79.8144)
  line L4 (-31, 79.8144) -> (-31, 71.8144)
  line L5 (-31, 79.8144) -> (-26, 79.8144) projected
  line L6 (-34, 79.8144) -> (-22, 79.8144) construction
  line L7 (-22, 79.8144) -> (-22, 111.8144) construction
  line L8 (-22, 111.8144) -> (-34, 111.8144) construction
  line L9 (-34, 111.8144) -> (-34, 79.8144) construction
  line L10 (-35, 76.8144) -> (-32, 76.8144)
  line L11 (-32, 76.8144) -> (-32, 79.8144)
  line L12 (-32, 79.8144) -> (-35, 79.8144)
  line L13 (-35, 79.8144) -> (-35, 76.8144)
  line L14 (-34, 89.8144) -> (-22, 89.8144) construction
  line L15 (-34, 89.8144) -> (-37, 89.8144)
  line L16 (-37, 89.8144) -> (-37, 92.8144)
  line L17 (-37, 92.8144) -> (-34, 92.8144)
  line L18 (-34, 92.8144) -> (-34, 89.8144)
  line L19 (-22, 89.8144) -> (-19, 89.8144)
  line L20 (-19, 89.8144) -> (-19, 92.8144)
  line L21 (-19, 92.8144) -> (-22, 92.8144)
  line L22 (-22, 92.8144) -> (-22, 89.8144)
  line L23 (-24, 76.8144) -> (-21, 76.8144)
  line L24 (-21, 76.8144) -> (-21, 79.8144)
  line L25 (-21, 79.8144) -> (-24, 79.8144)
  line L26 (-24, 79.8144) -> (-24, 76.8144)
  circle A0 centre (-36.5, 84.8144) radius 1.5
  circle A1 centre (-19.5, 84.8144) radius 1.5
  line L27 (-26, 101.8144) -> (-26, 135) projected
  line L28 (-26, 101.8144) -> (-21, 101.8144)
  line L29 (-21, 101.8144) -> (-21, 111.8144)
  line L30 (-21, 111.8144) -> (-26, 111.8144)
  line L31 (-26, 111.8144) -> (-26, 101.8144)
  point P0 (0, 0)
  point P1 (-28, 79.8144)
  point P2 (-28, 111.8144)
  point P3 (-34, 107.8144)
  point P4 (-22, 104.8144)
  point P5 (-19, 107.8144)
  point P6 (-26, 65.5022)
  dimension "d151" = 6
  dimension "d152" = 12
  dimension "d153" = 40
  dimension "d154" = 3
  dimension "d155" = 3
  dimension "d156" = 0
  dimension "d157" = 1
  dimension "d158" = 10
  dimension "d159" = 3
  dimension "d160" = 3
  dimension "d171" = 3
  dimension "d172" = 3
  dimension "d173" = 1
  dimension "d174" = 3
  dimension "d175" = 3
  dimension "d176" = 3
  dimension "d177" = 2.5
  dimension "d178" = 2.5
  dimension "d179" = 5
  dimension "d180" = 5
  dimension "d181" = 8
  dimension "d182" = 5
  dimension "d183" = 10
  constraints: 58 end point, 14 parallel, 8 perpendicular, 7 horizontal, 5 point on line, 4 collinear, 2 centre point, 2 midpoint, 1 vertical alignment
  measures "d151" distance between parallel lines of L2 L4
  measures "d152" distance between parallel lines of L7 L9
  measures "d153" distance between parallel lines of L8 L1
  measures "d154" distance of L12.end L10.start
  measures "d155" distance of L11.end L12.end
  measures "d156" distance between parallel lines of L6 L12
  measures "d157" distance between parallel lines of L9 L13
  measures "d158" distance between parallel lines of L6 L14
  measures "d159" distance of L15.end L16.end
  measures "d160" distance of L16.end L17.end
  measures "d171" distance of L23.start L23.end
  measures "d172" distance of L23.end L24.end
  measures "d173" distance between parallel lines of L7 L24
  measures "d174" distance of L14.end L19.end
  measures "d175" diameter of A0
  measures "d176" diameter of A1
  measures "d177" distance from line of L7 A1.centre
  measures "d178" distance from line of L9 A0.centre
  measures "d179" distance from line of L15 A0.centre
  measures "d180" distance from line of L19 A1.centre
  measures "d181" distance between parallel lines of L26 L11
  measures "d182" distance of L29.end L30.end
  measures "d183" distance of L28.end L29.end
extrude "擠出16" cut sketch "草圖24" against normal up to surface (3 mm away) contours L13 L12 L11 L10 | L15 L16 L17 L18 | L22 L21 L20 L19 | L26 L25 L24 L23 | A0 | A1 | L27 L30 L29 L28
ref_plane "工作平面1" through (-10.5456, 0, -145) normal (0, 0, -1) x (-1, 0, 0)
mirror "鏡射1" about plane through (-10.5456, 0, -145) normal (0, 0, -1) of "擠出15", "擠出16"
sketch "草圖25" plane through (0, 3, 0) normal (0, 1, 0) x (1, 0, 0)
  line L0 (-34.1, 141) -> (-37, 141) projected
  line L1 (-37, 141) -> (-37, 149) projected
  line L2 (-37, 149) -> (-34.1, 149) projected
  line L3 (-34.1, 149) -> (-34.1, 141) projected
  line L4 (-26, 31) -> (-26, 79.8144) projected
  line L5 (-26, 111.8144) -> (-26, 135) projected
  arc A0 (-26, 31) -> (-28.1031, 26.625) centre (-16, 23.5) ccw projected
  arc A1 (-28.1031, 26.625) -> (-27.619, 26) centre (-27.619, 26.5) ccw projected
  line L6 (-27.619, 26) -> (-21.7663, 26) projected
  arc A2 (-21.7663, 26) -> (-21.3227, 26.2692) centre (-21.7663, 26.5) ccw projected
  arc A3 (-21.3227, 20.7308) -> (-21.3227, 26.2692) centre (-16, 23.5) ccw projected
  arc A4 (-21.3227, 20.7308) -> (-21.7663, 21) centre (-21.7663, 20.5) ccw projected
  line L7 (-21.7663, 21) -> (-27.619, 21) projected
  arc A5 (-27.619, 21) -> (-28.1031, 20.375) centre (-27.619, 20.5) ccw projected
  arc A6 (-28.1031, 20.375) -> (-26, 16) centre (-16, 23.5) ccw projected
  line L8 (-26, 3) -> (-26, 16) projected
  line L9 (-20, 3) -> (-26, 3) projected
  line L10 (-20, 3) -> (-20, 0) projected
  line L11 (-20, 0) -> (-14, 0) projected
  line L12 (-14, 0) -> (-14, 3) projected
  line L13 (-14, 3) -> (-6, 3) projected
  line L14 (-6, 3) -> (-6, 142.5) projected
  line L15 (-6, 142.5) -> (-10.5456, 142.5) projected
  arc A7 (-10.5456, 147.5) -> (-10.5456, 142.5) centre (-16, 145) ccw projected
  line L16 (-10.5456, 147.5) -> (-6, 147.5) projected
  line L17 (-6, 147.5) -> (-6, 287) projected
  line L18 (-6, 287) -> (-14, 287) projected
  line L19 (-14, 287) -> (-14, 290) projected
  line L20 (-14, 290) -> (-20, 290) projected
  line L21 (-20, 290) -> (-20, 287) projected
  line L22 (-26, 287) -> (-20, 287) projected
  line L23 (-26, 274) -> (-26, 287) projected
  arc A8 (-26, 274) -> (-28.1031, 269.625) centre (-16, 266.5) ccw projected
  arc A9 (-28.1031, 269.625) -> (-27.619, 269) centre (-27.619, 269.5) ccw projected
  line L24 (-27.619, 269) -> (-21.7663, 269) projected
  arc A10 (-21.7663, 269) -> (-21.3227, 269.2692) centre (-21.7663, 269.5) ccw projected
  arc A11 (-21.3227, 263.7308) -> (-21.3227, 269.2692) centre (-16, 266.5) ccw projected
  arc A12 (-21.3227, 263.7308) -> (-21.7663, 264) centre (-21.7663, 263.5) ccw projected
  line L25 (-21.7663, 264) -> (-27.619, 264) projected
  arc A13 (-27.619, 264) -> (-28.1031, 263.375) centre (-27.619, 263.5) ccw projected
  arc A14 (-28.1031, 263.375) -> (-26, 259) centre (-16, 266.5) ccw projected
  line L26 (-26, 155) -> (-26, 178.1856) projected
  line L27 (-26, 210.1856) -> (-26, 259) projected
  line L28 (-26, 155) -> (-41, 155) projected
  line L29 (-41, 155) -> (-41, 135) projected
  line L30 (-41, 135) -> (-26, 135) projected
  line L31 (-22.9, 239) -> (-20, 239) projected
  line L32 (-20, 239) -> (-20, 231) projected
  line L33 (-20, 231) -> (-22.9, 231) projected
  line L34 (-22.9, 231) -> (-22.9, 239) projected
  line L35 (-22.9, 59) -> (-20, 59) projected
  line L36 (-20, 59) -> (-20, 51) projected
  line L37 (-20, 51) -> (-22.9, 51) projected
  line L38 (-22.9, 51) -> (-22.9, 59) projected
  circle A15 centre (-16, 153.5) radius 1.5 projected
  circle A16 centre (-16, 136.5) radius 1.5 projected
  line L39 (-8, 231) -> (-11, 231) projected
  line L40 (-11, 231) -> (-11, 239) projected
  line L41 (-11, 239) -> (-8, 239) projected
  line L42 (-8, 239) -> (-8, 231) projected
  line L43 (-8, 286) -> (-8, 280) projected
  line L44 (-8, 280) -> (-11, 280) projected
  line L45 (-11, 280) -> (-11, 286) projected
  line L46 (-11, 286) -> (-8, 286) projected
  line L47 (-8, 51) -> (-11, 51) projected
  line L48 (-11, 51) -> (-11, 59) projected
  line L49 (-11, 59) -> (-8, 59) projected
  line L50 (-8, 59) -> (-8, 51) projected
  line L51 (-8, 10) -> (-8, 4) projected
  line L52 (-8, 4) -> (-11, 4) projected
  line L53 (-11, 4) -> (-11, 10) projected
  line L54 (-11, 10) -> (-8, 10) projected
  circle A17 centre (-16, 15) radius 1.5 projected
  circle A18 centre (-16, 275) radius 1.5 projected
  circle A19 centre (-16, 258) radius 1.5 projected
  circle A20 centre (-16, 32) radius 1.5 projected
  line L55 (-21, 178.1856) -> (-26, 178.1856) projected
  line L56 (-26, 111.8144) -> (-21, 111.8144) projected
  line L57 (-21, 111.8144) -> (-21, 101.8144) projected
  line L58 (-21, 101.8144) -> (-42.4222, 101.8144) projected
  line L59 (-42.4222, 101.8144) -> (-42.4222, 71.8144) projected
  line L60 (-42.4222, 71.8144) -> (-31, 71.8144) projected
  line L61 (-31, 71.8144) -> (-31, 79.8144) projected
  line L62 (-31, 79.8144) -> (-26, 79.8144) projected
  line L63 (-31, 210.1856) -> (-26, 210.1856) projected
  line L64 (-31, 218.1856) -> (-31, 210.1856) projected
  line L65 (-42.4222, 218.1856) -> (-31, 218.1856) projected
  line L66 (-42.4222, 188.1856) -> (-42.4222, 218.1856) projected
  line L67 (-42.4222, 188.1856) -> (-21, 188.1856) projected
  line L68 (-21, 188.1856) -> (-21, 178.1856) projected
  point P0 (0, 0)
sketch "草圖26" plane through (0, 3, 0) normal (0, 1, 0) x (1, 0, 0)
  line L0 (-21, 178.1856) -> (-26, 178.1856) projected
  line L1 (-26, 155) -> (-26, 178.1856) projected
  line L2 (-26, 155) -> (-41, 155) projected
  line L3 (-41, 155) -> (-41, 135) projected
  line L4 (-41, 135) -> (-26, 135) projected
  line L5 (-26, 111.8144) -> (-26, 135) projected
  line L6 (-26, 111.8144) -> (-21, 111.8144) projected
  line L7 (-21, 111.8144) -> (-21, 101.8144) projected
  line L8 (-21, 101.8144) -> (-42.4222, 101.8144) projected
  line L9 (-42.4222, 101.8144) -> (-42.4222, 71.8144) projected
  line L10 (-42.4222, 71.8144) -> (-31, 71.8144) projected
  line L11 (-31, 71.8144) -> (-31, 79.8144) projected
  line L12 (-31, 79.8144) -> (-26, 79.8144) projected
  line L13 (-26, 31) -> (-26, 79.8144) projected
  arc A0 (-26, 31) -> (-28.1031, 26.625) centre (-16, 23.5) ccw projected
  arc A1 (-28.1031, 26.625) -> (-27.619, 26) centre (-27.619, 26.5) ccw projected
  line L14 (-27.619, 26) -> (-21.7663, 26) projected
  arc A2 (-21.7663, 26) -> (-21.3227, 26.2692) centre (-21.7663, 26.5) ccw projected
  arc A3 (-21.3227, 20.7308) -> (-21.3227, 26.2692) centre (-16, 23.5) ccw projected
  arc A4 (-21.3227, 20.7308) -> (-21.7663, 21) centre (-21.7663, 20.5) ccw projected
  line L15 (-21.7663, 21) -> (-27.619, 21) projected
  arc A5 (-27.619, 21) -> (-28.1031, 20.375) centre (-27.619, 20.5) ccw projected
  arc A6 (-28.1031, 20.375) -> (-26, 16) centre (-16, 23.5) ccw projected
  line L16 (-26, 3) -> (-26, 16) projected
  line L17 (-20, 3) -> (-26, 3) projected
  line L18 (-20, 3) -> (-20, 0) projected
  line L19 (-20, 0) -> (-14, 0) projected
  line L20 (-14, 0) -> (-14, 3) projected
  line L21 (-14, 3) -> (-6, 3) projected
  line L22 (-6, 3) -> (-6, 142.5) projected
  line L23 (-6, 142.5) -> (-10.5456, 142.5) projected
  arc A7 (-10.5456, 147.5) -> (-10.5456, 142.5) centre (-16, 145) ccw projected
  line L24 (-10.5456, 147.5) -> (-6, 147.5) projected
  line L25 (-6, 147.5) -> (-6, 287) projected
  line L26 (-6, 287) -> (-14, 287) projected
  line L27 (-14, 287) -> (-14, 290) projected
  line L28 (-14, 290) -> (-20, 290) projected
  line L29 (-20, 290) -> (-20, 287) projected
  line L30 (-26, 287) -> (-20, 287) projected
  line L31 (-26, 274) -> (-26, 287) projected
  arc A8 (-26, 274) -> (-28.1031, 269.625) centre (-16, 266.5) ccw projected
  arc A9 (-28.1031, 269.625) -> (-27.619, 269) centre (-27.619, 269.5) ccw projected
  line L32 (-27.619, 269) -> (-21.7663, 269) projected
  arc A10 (-21.7663, 269) -> (-21.3227, 269.2692) centre (-21.7663, 269.5) ccw projected
  arc A11 (-21.3227, 263.7308) -> (-21.3227, 269.2692) centre (-16, 266.5) ccw projected
  arc A12 (-21.3227, 263.7308) -> (-21.7663, 264) centre (-21.7663, 263.5) ccw projected
  line L33 (-21.7663, 264) -> (-27.619, 264) projected
  arc A13 (-27.619, 264) -> (-28.1031, 263.375) centre (-27.619, 263.5) ccw projected
  arc A14 (-28.1031, 263.375) -> (-26, 259) centre (-16, 266.5) ccw projected
  line L34 (-26, 210.1856) -> (-26, 259) projected
  line L35 (-31, 210.1856) -> (-26, 210.1856) projected
  line L36 (-31, 218.1856) -> (-31, 210.1856) projected
  line L37 (-42.4222, 218.1856) -> (-31, 218.1856) projected
  line L38 (-42.4222, 188.1856) -> (-42.4222, 218.1856) projected
  line L39 (-42.4222, 188.1856) -> (-21, 188.1856) projected
  line L40 (-21, 188.1856) -> (-21, 178.1856) projected
  circle A15 centre (-19.5, 205.1856) radius 1.5 projected
  line L41 (-35, 213.1856) -> (-32, 213.1856) projected
  line L42 (-32, 213.1856) -> (-32, 210.1856) projected
  line L43 (-32, 210.1856) -> (-35, 210.1856) projected
  line L44 (-35, 210.1856) -> (-35, 213.1856) projected
  line L45 (-19, 200.1856) -> (-19, 197.1856) projected
  line L46 (-19, 197.1856) -> (-22, 197.1856) projected
  line L47 (-22, 197.1856) -> (-22, 200.1856) projected
  line L48 (-22, 200.1856) -> (-19, 200.1856) projected
  line L49 (-24, 213.1856) -> (-21, 213.1856) projected
  line L50 (-21, 213.1856) -> (-21, 210.1856) projected
  line L51 (-21, 210.1856) -> (-24, 210.1856) projected
  line L52 (-24, 210.1856) -> (-24, 213.1856) projected
  circle A16 centre (-36.5, 205.1856) radius 1.5 projected
  line L53 (-34, 200.1856) -> (-34, 197.1856) projected
  line L54 (-34, 197.1856) -> (-37, 197.1856) projected
  line L55 (-37, 197.1856) -> (-37, 200.1856) projected
  line L56 (-37, 200.1856) -> (-34, 200.1856) projected
  line L57 (-34.1, 141) -> (-37, 141) projected
  line L58 (-37, 141) -> (-37, 149) projected
  line L59 (-37, 149) -> (-34.1, 149) projected
  line L60 (-34.1, 149) -> (-34.1, 141) projected
  line L61 (-22.9, 239) -> (-20, 239) projected
  line L62 (-20, 239) -> (-20, 231) projected
  line L63 (-20, 231) -> (-22.9, 231) projected
  line L64 (-22.9, 231) -> (-22.9, 239) projected
  line L65 (-22.9, 59) -> (-20, 59) projected
  line L66 (-20, 59) -> (-20, 51) projected
  line L67 (-20, 51) -> (-22.9, 51) projected
  line L68 (-22.9, 51) -> (-22.9, 59) projected
  circle A17 centre (-16, 153.5) radius 1.5 projected
  circle A18 centre (-16, 136.5) radius 1.5 projected
  line L69 (-8, 231) -> (-11, 231) projected
  line L70 (-11, 231) -> (-11, 239) projected
  line L71 (-11, 239) -> (-8, 239) projected
  line L72 (-8, 239) -> (-8, 231) projected
  line L73 (-8, 286) -> (-8, 280) projected
  line L74 (-8, 280) -> (-11, 280) projected
  line L75 (-11, 280) -> (-11, 286) projected
  line L76 (-11, 286) -> (-8, 286) projected
  line L77 (-8, 51) -> (-11, 51) projected
  line L78 (-11, 51) -> (-11, 59) projected
  line L79 (-11, 59) -> (-8, 59) projected
  line L80 (-8, 59) -> (-8, 51) projected
  line L81 (-8, 10) -> (-8, 4) projected
  line L82 (-8, 4) -> (-11, 4) projected
  line L83 (-11, 4) -> (-11, 10) projected
  line L84 (-11, 10) -> (-8, 10) projected
  circle A19 centre (-16, 15) radius 1.5 projected
  circle A20 centre (-16, 275) radius 1.5 projected
  circle A21 centre (-16, 258) radius 1.5 projected
  circle A22 centre (-16, 32) radius 1.5 projected
  line L85 (-34, 92.8144) -> (-34, 89.8144) projected
  line L86 (-34, 89.8144) -> (-37, 89.8144) projected
  line L87 (-37, 89.8144) -> (-37, 92.8144) projected
  line L88 (-37, 92.8144) -> (-34, 92.8144) projected
  circle A23 centre (-36.5, 84.8144) radius 1.5 projected
  line L89 (-21, 76.8144) -> (-24, 76.8144) projected
  line L90 (-24, 76.8144) -> (-24, 79.8144) projected
  line L91 (-24, 79.8144) -> (-21, 79.8144) projected
  line L92 (-21, 79.8144) -> (-21, 76.8144) projected
  line L93 (-19, 92.8144) -> (-19, 89.8144) projected
  line L94 (-19, 89.8144) -> (-22, 89.8144) projected
  line L95 (-22, 89.8144) -> (-22, 92.8144) projected
  line L96 (-22, 92.8144) -> (-19, 92.8144) projected
  line L97 (-32, 76.8144) -> (-35, 76.8144) projected
  line L98 (-35, 76.8144) -> (-35, 79.8144) projected
  line L99 (-35, 79.8144) -> (-32, 79.8144) projected
  line L100 (-32, 79.8144) -> (-32, 76.8144) projected
  circle A24 centre (-19.5, 84.8144) radius 1.5 projected
  point P0 (0, 0)
equation "\"d8\" = 0.5 * d7"
equation "\"d35\" = 0.5 * d34"
equation "\"d31\" = d27"
equation "\"d58\" = d21"
equation "\"d59\" = d20"
equation "\"d60\" = d22"
equation "\"d44\" = 0.5 * d43"
equation "\"d48\" = 2 * d45"
